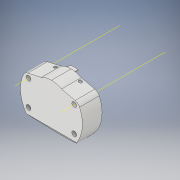
# Autodesk Inventor part: DGB_002_NewCover
Saved by Autodesk Inventor 2018 (Build 220112000, 112)
## iProperties
Created: 2020-01-12
Part Number: DGB_002_NewCover
Material: ABS Plastic
Document SubType Name: Modeling
Designer: user
Density: 1.06 g/cm^3
Appearance: Smooth - White
Mass: 38.8986 g
Surface Area: 471.13 cm^2
Volume: 36.6968 cm^3
Author: user
Autodesk Inventor part; units mm, degrees
ref_plane "YZ Plane" through (0, 0, 0) normal (1, 0, 0) x (0, 1, 0)
sketch "Sketch1" plane through (0, 0, 0) normal (0, 0, 1) x (1, 0, 0)
  line L0 (61.459706, -2.433337) -> (77.570916, 69.357275) construction
  arc A0 (77.570916, 69.357275) -> (52.904901, 108.47351) centre (45.600116, 76.532144) ccw construction
  line L1 (9.160225, 118.477636) -> (52.904901, 108.47351) construction
  arc A1 (9.160225, 118.477636) -> (-9.526433, 118.477636) centre (-0.183104, 77.6224) ccw construction
  line L2 (-9.526433, 118.477636) -> (-53.271109, 108.47351) construction
  arc A2 (-53.271109, 108.47351) -> (-77.937124, 69.357275) centre (-45.966325, 76.532144) ccw construction
  line L3 (-77.937124, 69.357275) -> (-61.825914, -2.433337) construction
  arc A3 (-61.825914, -2.433337) -> (-56.608807, -9.583273) centre (-50.983104, 0) ccw construction
  line L4 (-56.608807, -9.583273) -> (-18.828292, -31.761705) construction
  arc A4 (-18.828292, -31.761705) -> (18.462083, -31.761705) centre (-0.183104, 0) ccw construction
  line L5 (56.242599, -9.583273) -> (18.462083, -31.761705) construction
  arc A5 (56.242599, -9.583273) -> (61.459706, -2.433337) centre (50.616896, 0) ccw construction
  circle A6 centre (0, 41.9862) radius 14.2875 construction
  circle A7 centre (0, 77.6224) radius 14.2875 construction
  circle A8 centre (45.78322, 76.532144) radius 9.5631 construction
  circle A9 centre (23.8125, 0) radius 2.0193 construction
  circle A10 centre (-23.8125, 0) radius 2.0193 construction
  circle A11 centre (15.947858, 9.2075) radius 2.0193 construction
  circle A12 centre (-15.947858, 9.2075) radius 2.0193 construction
  circle A13 centre (0, -18.415) radius 2.0193 construction
  circle A14 centre (-45.78322, 51.132144) radius 2.4892 construction
  circle A15 centre (-45.78322, 101.932144) radius 2.4892 construction
  circle A16 centre (45.78322, 101.932144) radius 2.4892 construction
  circle A17 centre (45.78322, 51.132144) radius 2.4892 construction
  circle A18 centre (50.8, 0) radius 9.5758 construction
  circle A19 centre (-50.8, 0) radius 9.5758 construction
  line L6 (-3.175, 99.337246) -> (-3.175, 109.347752) construction
  arc A20 (-5.473828, 96.26646) -> (-3.175, 99.337246) centre (-6.3754, 99.337246) ccw construction
  arc A21 (-5.473828, 96.26646) -> (-18.769089, 82.650824) centre (0, 77.6224) ccw construction
  arc A22 (-21.784278, 80.279542) -> (-18.769089, 82.650824) centre (-21.860469, 83.479034) ccw construction
  line L7 (-21.784278, 80.279542) -> (-27.885438, 80.134252) construction
  arc A23 (-30.95167, 82.192597) -> (-27.885438, 80.134252) centre (-27.961629, 83.333745) ccw construction
  arc A24 (-30.95167, 82.192597) -> (-40.477461, 91.494248) centre (-45.78322, 76.532144) ccw construction
  arc A25 (-42.60822, 94.510608) -> (-40.477461, 91.494248) centre (-39.40782, 94.510608) ccw construction
  line L8 (-42.60822, 94.510608) -> (-42.60822, 95.929379) construction
  arc A26 (-41.737916, 98.123283) -> (-42.60822, 95.929379) centre (-39.40782, 95.929379) ccw construction
  arc A27 (-41.737916, 98.123283) -> (-40.233223, 102.195657) centre (-45.78322, 101.932144) ccw construction
  arc A28 (-37.749915, 105.467294) -> (-40.233223, 102.195657) centre (-37.036424, 102.34744) ccw construction
  line L9 (-7.927673, 112.287449) -> (-37.749915, 105.467294) construction
  arc A29 (-7.005934, 112.485425) -> (-7.927673, 112.287449) centre (0, 77.6224) ccw construction
  arc A30 (-3.175, 109.347752) -> (-7.005934, 112.485425) centre (-6.3754, 109.347752) ccw construction
  arc A31 (-54.866106, 101.337511) -> (-71.349124, 83.179673) centre (-45.78322, 76.532144) ccw construction
  arc A32 (-50.848233, 99.647945) -> (-54.866106, 101.337511) centre (-53.765679, 98.332246) ccw construction
  arc A33 (-50.848233, 99.647945) -> (-49.828525, 98.123283) centre (-45.78322, 101.932144) ccw construction
  arc A34 (-48.95822, 95.929379) -> (-49.828525, 98.123283) centre (-52.15862, 95.929379) ccw construction
  line L10 (-48.95822, 94.510608) -> (-48.95822, 95.929379) construction
  arc A35 (-51.088979, 91.494248) -> (-48.95822, 94.510608) centre (-52.15862, 94.510608) ccw construction
  arc A36 (-51.088979, 91.494248) -> (-60.867396, 81.480201) centre (-45.78322, 76.532144) ccw construction
  arc A37 (-63.832175, 79.278237) -> (-60.867396, 81.480201) centre (-63.908366, 82.477729) ccw construction
  line L11 (-63.832175, 79.278237) -> (-68.175525, 79.174806) construction
  arc A38 (-71.349124, 83.179673) -> (-68.175525, 79.174806) centre (-68.251716, 82.374299) ccw construction
  line L12 (-63.681003, 72.930036) -> (-68.102406, 72.824747) construction
  arc A39 (-60.614771, 70.871691) -> (-63.681003, 72.930036) centre (-63.604812, 69.730543) ccw construction
  arc A40 (-60.614771, 70.871691) -> (-51.088979, 61.57004) centre (-45.78322, 76.532144) ccw construction
  arc A41 (-48.95822, 58.55368) -> (-51.088979, 61.57004) centre (-52.15862, 58.55368) ccw construction
  line L13 (-48.95822, 57.13491) -> (-48.95822, 58.55368) construction
  arc A42 (-49.828525, 54.941005) -> (-48.95822, 57.13491) centre (-52.15862, 57.13491) ccw construction
  arc A43 (-49.828525, 54.941005) -> (-51.248421, 52.133894) centre (-45.78322, 51.132144) ccw construction
  arc A44 (-52.500008, 50.13285) -> (-51.248421, 52.133894) centre (-54.396376, 52.710901) ccw construction
  line L14 (-52.500008, 50.13285) -> (-60.545848, 44.214475) construction
  arc A45 (-62.828817, 43.615562) -> (-60.545848, 44.214475) centre (-62.442216, 46.792526) ccw construction
  arc A46 (-62.828817, 43.615562) -> (-63.126943, 43.643712) centre (-63.5, 38.1) ccw construction
  arc A47 (-66.034792, 46.136089) -> (-63.126943, 43.643712) centre (-62.912063, 46.83689) ccw construction
  line L15 (-71.148944, 68.924453) -> (-66.034792, 46.136089) construction
  arc A48 (-68.102406, 72.824747) -> (-71.148944, 68.924453) centre (-68.026215, 69.625254) ccw construction
  line L16 (-40.941493, -11.309739) -> (-15.4305, -26.285549) construction
  arc A49 (-41.887958, -6.63801) -> (-40.941493, -11.309739) centre (-39.32129, -8.549756) ccw construction
  arc A50 (-41.887958, -6.63801) -> (-40.850794, -4.949845) centre (-50.8, 0) ccw construction
  arc A51 (-37.985423, -3.175) -> (-40.850794, -4.949845) centre (-37.985423, -6.3754) ccw construction
  line L17 (-29.815266, -3.175) -> (-37.985423, -3.175) construction
  arc A52 (-27.621361, -4.045305) -> (-29.815266, -3.175) centre (-29.815266, -6.3754) ccw construction
  arc A53 (-27.621361, -4.045305) -> (-21.832221, -5.191378) centre (-23.8125, 0) ccw construction
  arc A54 (-17.715395, -7.004805) -> (-21.832221, -5.191378) centre (-20.691581, -8.181612) ccw construction
  arc A55 (-17.715395, -7.004805) -> (-7.267025, -17.609453) centre (0, 0) ccw construction
  arc A56 (-5.385714, -19.781016) -> (-7.267025, -17.609453) centre (-8.487885, -20.567842) ccw construction
  arc A57 (-5.385714, -19.781016) -> (-4.045305, -22.223861) centre (0, -18.415) ccw construction
  arc A58 (-3.175, -24.417766) -> (-4.045305, -22.223861) centre (-6.3754, -24.417766) ccw construction
  line L18 (-3.175, -26.524156) -> (-3.175, -24.417766) construction
  arc A59 (-7.123352, -29.635928) -> (-3.175, -26.524156) centre (-6.3754, -26.524156) ccw construction
  arc A60 (-15.4305, -26.285549) -> (-7.123352, -29.635928) centre (0, 0) ccw construction
  arc A61 (18.769089, 82.650824) -> (5.473828, 96.26646) centre (0, 77.6224) ccw construction
  arc A62 (3.175, 99.337246) -> (5.473828, 96.26646) centre (6.3754, 99.337246) ccw construction
  line L19 (3.175, 99.337246) -> (3.175, 109.347752) construction
  arc A63 (7.005934, 112.485425) -> (3.175, 109.347752) centre (6.3754, 109.347752) ccw construction
  arc A64 (7.927673, 112.287449) -> (7.005934, 112.485425) centre (0, 77.6224) ccw construction
  line L20 (7.927673, 112.287449) -> (37.749915, 105.467294) construction
  arc A65 (40.233223, 102.195657) -> (37.749915, 105.467294) centre (37.036424, 102.34744) ccw construction
  arc A66 (40.233223, 102.195657) -> (41.737916, 98.123283) centre (45.78322, 101.932144) ccw construction
  arc A67 (42.60822, 95.929379) -> (41.737916, 98.123283) centre (39.40782, 95.929379) ccw construction
  line L21 (42.60822, 94.510608) -> (42.60822, 95.929379) construction
  arc A68 (40.477461, 91.494248) -> (42.60822, 94.510608) centre (39.40782, 94.510608) ccw construction
  arc A69 (40.477461, 91.494248) -> (30.95167, 82.192597) centre (45.78322, 76.532144) ccw construction
  arc A70 (27.885438, 80.134252) -> (30.95167, 82.192597) centre (27.961629, 83.333745) ccw construction
  line L22 (21.784278, 80.279542) -> (27.885438, 80.134252) construction
  arc A71 (18.769089, 82.650824) -> (21.784278, 80.279542) centre (21.860469, 83.479034) ccw construction
  arc A72 (49.828525, 98.123283) -> (50.848233, 99.647945) centre (45.78322, 101.932144) ccw construction
  arc A73 (54.866106, 101.337511) -> (50.848233, 99.647945) centre (53.765679, 98.332246) ccw construction
  arc A74 (71.349124, 83.179673) -> (54.866106, 101.337511) centre (45.78322, 76.532144) ccw construction
  arc A75 (68.175525, 79.174806) -> (71.349124, 83.179673) centre (68.251716, 82.374299) ccw construction
  line L23 (63.832175, 79.278237) -> (68.175525, 79.174806) construction
  arc A76 (60.867396, 81.480201) -> (63.832175, 79.278237) centre (63.908366, 82.477729) ccw construction
  arc A77 (60.867396, 81.480201) -> (51.088979, 91.494248) centre (45.78322, 76.532144) ccw construction
  arc A78 (48.95822, 94.510608) -> (51.088979, 91.494248) centre (52.15862, 94.510608) ccw construction
  line L24 (48.95822, 94.510608) -> (48.95822, 95.929379) construction
  arc A79 (49.828525, 98.123283) -> (48.95822, 95.929379) centre (52.15862, 95.929379) ccw construction
  arc A80 (54.402179, 10.512467) -> (49.473378, 11.033029) centre (50.8, 0) ccw construction
  arc A81 (46.416616, 12.45311) -> (49.473378, 11.033029) centre (49.091311, 14.210541) ccw construction
  line L25 (46.416616, 12.45311) -> (28.364069, 39.927902) construction
  arc A82 (30.411819, 44.823724) -> (28.364069, 39.927902) centre (31.038764, 41.685333) ccw construction
  line L26 (30.411819, 44.823724) -> (40.518729, 46.842744) construction
  arc A83 (42.840615, 46.419079) -> (40.518729, 46.842744) centre (41.145674, 43.704353) ccw construction
  arc A84 (42.840615, 46.419079) -> (46.454403, 45.616582) centre (45.78322, 51.132144) ccw construction
  arc A85 (48.737373, 45.017669) -> (46.454403, 45.616582) centre (46.841005, 42.439618) ccw construction
  line L27 (48.737373, 45.017669) -> (56.783213, 39.099294) construction
  arc A86 (58.0348, 37.09825) -> (56.783213, 39.099294) centre (54.886845, 36.521243) ccw construction
  arc A87 (58.0348, 37.09825) -> (60.793794, 33.247334) centre (63.5, 38.1) ccw construction
  arc A88 (62.357749, 29.751398) -> (60.793794, 33.247334) centre (59.23502, 30.452199) ccw construction
  line L28 (62.357749, 29.751398) -> (58.562335, 12.839257) construction
  arc A89 (54.402179, 10.512467) -> (58.562335, 12.839257) centre (55.439606, 13.540058) ccw construction
  arc A90 (12.787451, 62.992128) -> (12.738922, 56.150322) centre (15.796264, 59.549712) ccw construction
  arc A91 (12.787451, 62.992128) -> (18.508462, 71.70627) centre (0, 77.6224) ccw construction
  arc A92 (21.633105, 73.931341) -> (18.508462, 71.70627) centre (21.556915, 70.731848) ccw construction
  line L29 (21.633105, 73.931341) -> (27.734266, 73.786052) construction
  arc A93 (30.699045, 71.584087) -> (27.734266, 73.786052) centre (27.658075, 70.586559) ccw construction
  arc A94 (30.699045, 71.584087) -> (40.477461, 61.57004) centre (45.78322, 76.532144) ccw construction
  arc A95 (42.60822, 58.55368) -> (40.477461, 61.57004) centre (39.40782, 58.55368) ccw construction
  line L30 (42.60822, 57.13491) -> (42.60822, 58.55368) construction
  arc A96 (41.737916, 54.941005) -> (42.60822, 57.13491) centre (39.40782, 57.13491) ccw construction
  arc A97 (41.737916, 54.941005) -> (41.255699, 54.35293) centre (45.78322, 51.132144) ccw construction
  arc A98 (39.274791, 53.069711) -> (41.255699, 54.35293) centre (38.647846, 56.208103) ccw construction
  line L31 (20.28247, 49.275686) -> (39.274791, 53.069711) construction
  arc A99 (16.828361, 50.914177) -> (20.28247, 49.275686) centre (19.655525, 52.414077) ccw construction
  arc A100 (16.828361, 50.914177) -> (12.738922, 56.150322) centre (0, 41.9862) ccw construction
  arc A101 (40.850794, -4.949845) -> (41.887958, -6.63801) centre (50.8, 0) ccw construction
  arc A102 (40.941493, -11.309739) -> (41.887958, -6.63801) centre (39.32129, -8.549756) ccw construction
  line L32 (40.941493, -11.309739) -> (15.4305, -26.285549) construction
  arc A103 (7.123352, -29.635928) -> (15.4305, -26.285549) centre (0, 0) ccw construction
  arc A104 (3.175, -26.524156) -> (7.123352, -29.635928) centre (6.3754, -26.524156) ccw construction
  line L33 (3.175, -26.524156) -> (3.175, -24.417766) construction
  arc A105 (4.045305, -22.223861) -> (3.175, -24.417766) centre (6.3754, -24.417766) ccw construction
  arc A106 (4.045305, -22.223861) -> (5.385714, -19.781016) centre (0, -18.415) ccw construction
  arc A107 (7.267025, -17.609453) -> (5.385714, -19.781016) centre (8.487885, -20.567842) ccw construction
  arc A108 (7.267025, -17.609453) -> (17.715395, -7.004805) centre (0, 0) ccw construction
  arc A109 (21.832221, -5.191378) -> (17.715395, -7.004805) centre (20.691581, -8.181612) ccw construction
  arc A110 (21.832221, -5.191378) -> (27.621361, -4.045305) centre (23.8125, 0) ccw construction
  arc A111 (29.815266, -3.175) -> (27.621361, -4.045305) centre (29.815266, -6.3754) ccw construction
  line L34 (29.815266, -3.175) -> (37.985423, -3.175) construction
  arc A112 (40.850794, -4.949845) -> (37.985423, -3.175) centre (37.985423, -6.3754) ccw construction
  arc A113 (51.088979, 61.57004) -> (60.614771, 70.871691) centre (45.78322, 76.532144) ccw construction
  arc A114 (63.681003, 72.930036) -> (60.614771, 70.871691) centre (63.604812, 69.730543) ccw construction
  line L35 (63.681003, 72.930036) -> (68.102406, 72.824747) construction
  arc A115 (71.148944, 68.924453) -> (68.102406, 72.824747) centre (68.026215, 69.625254) ccw construction
  line L36 (71.148944, 68.924453) -> (66.034792, 46.136089) construction
  arc A116 (63.126943, 43.643712) -> (66.034792, 46.136089) centre (62.912063, 46.83689) ccw construction
  arc A117 (63.126943, 43.643712) -> (62.828817, 43.615562) centre (63.5, 38.1) ccw construction
  arc A118 (60.545848, 44.214475) -> (62.828817, 43.615562) centre (62.442216, 46.792526) ccw construction
  line L37 (52.500008, 50.13285) -> (60.545848, 44.214475) construction
  arc A119 (51.248421, 52.133894) -> (52.500008, 50.13285) centre (54.396376, 52.710901) ccw construction
  arc A120 (51.248421, 52.133894) -> (49.828525, 54.941005) centre (45.78322, 51.132144) ccw construction
  arc A121 (48.95822, 57.13491) -> (49.828525, 54.941005) centre (52.15862, 57.13491) ccw construction
  line L38 (48.95822, 57.13491) -> (48.95822, 58.55368) construction
  arc A122 (51.088979, 61.57004) -> (48.95822, 58.55368) centre (52.15862, 58.55368) ccw construction
  arc A123 (11.616722, 15.098155) -> (8.733861, 16.929919) centre (0, 0) ccw construction
  arc A124 (8.733861, 25.056281) -> (8.733861, 16.929919) centre (10.829988, 20.9931) ccw construction
  arc A125 (8.733861, 25.056281) -> (17.800734, 35.201189) centre (0, 41.9862) ccw construction
  arc A126 (23.465953, 35.818739) -> (17.800734, 35.201189) centre (20.791257, 34.061308) ccw construction
  line L39 (41.109681, 8.966143) -> (23.465953, 35.818739) construction
  arc A127 (41.199833, 5.596826) -> (41.109681, 8.966143) centre (38.434985, 7.208711) ccw construction
  arc A128 (41.199833, 5.596826) -> (40.850794, 4.949845) centre (50.8, 0) ccw construction
  arc A129 (37.985423, 3.175) -> (40.850794, 4.949845) centre (37.985423, 6.3754) ccw construction
  line L40 (29.815266, 3.175) -> (37.985423, 3.175) construction
  arc A130 (27.621361, 4.045305) -> (29.815266, 3.175) centre (29.815266, 6.3754) ccw construction
  arc A131 (27.621361, 4.045305) -> (24.369611, 5.528249) centre (23.8125, 0) ccw construction
  arc A132 (21.495224, 8.893427) -> (24.369611, 5.528249) centre (24.690507, 8.712521) ccw construction
  arc A133 (21.495224, 8.893427) -> (14.438006, 14.554673) centre (15.947858, 9.2075) ccw construction
  arc A134 (11.616722, 15.098155) -> (14.438006, 14.554673) centre (13.568331, 17.634645) ccw construction
  line L41 (-21.633105, 73.931341) -> (-27.734266, 73.786052) construction
  arc A135 (-18.508462, 71.70627) -> (-21.633105, 73.931341) centre (-21.556915, 70.731848) ccw construction
  arc A136 (-18.508462, 71.70627) -> (-12.787451, 62.992128) centre (0, 77.6224) ccw construction
  arc A137 (-12.738922, 56.150322) -> (-12.787451, 62.992128) centre (-15.796264, 59.549712) ccw construction
  arc A138 (-12.738922, 56.150322) -> (-16.828361, 50.914177) centre (0, 41.9862) ccw construction
  arc A139 (-20.28247, 49.275686) -> (-16.828361, 50.914177) centre (-19.655525, 52.414077) ccw construction
  line L42 (-20.28247, 49.275686) -> (-39.274791, 53.069711) construction
  arc A140 (-41.255699, 54.35293) -> (-39.274791, 53.069711) centre (-38.647846, 56.208103) ccw construction
  arc A141 (-41.255699, 54.35293) -> (-41.737916, 54.941005) centre (-45.78322, 51.132144) ccw construction
  arc A142 (-42.60822, 57.13491) -> (-41.737916, 54.941005) centre (-39.40782, 57.13491) ccw construction
  line L43 (-42.60822, 57.13491) -> (-42.60822, 58.55368) construction
  arc A143 (-40.477461, 61.57004) -> (-42.60822, 58.55368) centre (-39.40782, 58.55368) ccw construction
  arc A144 (-40.477461, 61.57004) -> (-30.699045, 71.584087) centre (-45.78322, 76.532144) ccw construction
  arc A145 (-27.734266, 73.786052) -> (-30.699045, 71.584087) centre (-27.658075, 70.586559) ccw construction
  arc A146 (-8.733861, 16.929919) -> (-8.733861, 25.056281) centre (-10.829988, 20.9931) ccw construction
  arc A147 (-8.733861, 16.929919) -> (-11.616722, 15.098155) centre (0, 0) ccw construction
  arc A148 (-14.438006, 14.554673) -> (-11.616722, 15.098155) centre (-13.568331, 17.634645) ccw construction
  arc A149 (-14.438006, 14.554673) -> (-21.495224, 8.893427) centre (-15.947858, 9.2075) ccw construction
  arc A150 (-24.369611, 5.528249) -> (-21.495224, 8.893427) centre (-24.690507, 8.712521) ccw construction
  arc A151 (-24.369611, 5.528249) -> (-27.621361, 4.045305) centre (-23.8125, 0) ccw construction
  arc A152 (-29.815266, 3.175) -> (-27.621361, 4.045305) centre (-29.815266, 6.3754) ccw construction
  line L44 (-29.815266, 3.175) -> (-37.985423, 3.175) construction
  arc A153 (-40.850794, 4.949845) -> (-37.985423, 3.175) centre (-37.985423, 6.3754) ccw construction
  arc A154 (-40.850794, 4.949845) -> (-41.199833, 5.596826) centre (-50.8, 0) ccw construction
  arc A155 (-41.109681, 8.966143) -> (-41.199833, 5.596826) centre (-38.434985, 7.208711) ccw construction
  line L45 (-41.109681, 8.966143) -> (-23.465953, 35.818739) construction
  arc A156 (-17.800734, 35.201189) -> (-23.465953, 35.818739) centre (-20.791257, 34.061308) ccw construction
  arc A157 (-17.800734, 35.201189) -> (-8.733861, 25.056281) centre (0, 41.9862) ccw construction
  line L46 (-46.416616, 12.45311) -> (-28.364069, 39.927902) construction
  arc A158 (-49.473378, 11.033029) -> (-46.416616, 12.45311) centre (-49.091311, 14.210541) ccw construction
  arc A159 (-49.473378, 11.033029) -> (-54.402179, 10.512467) centre (-50.8, 0) ccw construction
  arc A160 (-58.562335, 12.839257) -> (-54.402179, 10.512467) centre (-55.439606, 13.540058) ccw construction
  line L47 (-62.357749, 29.751398) -> (-58.562335, 12.839257) construction
  arc A161 (-60.793794, 33.247334) -> (-62.357749, 29.751398) centre (-59.23502, 30.452199) ccw construction
  arc A162 (-60.793794, 33.247334) -> (-58.0348, 37.09825) centre (-63.5, 38.1) ccw construction
  arc A163 (-56.783213, 39.099294) -> (-58.0348, 37.09825) centre (-54.886845, 36.521243) ccw construction
  line L48 (-48.737373, 45.017669) -> (-56.783213, 39.099294) construction
  arc A164 (-46.454403, 45.616582) -> (-48.737373, 45.017669) centre (-46.841005, 42.439618) ccw construction
  arc A165 (-46.454403, 45.616582) -> (-42.840615, 46.419079) centre (-45.78322, 51.132144) ccw construction
  arc A166 (-40.518729, 46.842744) -> (-42.840615, 46.419079) centre (-41.145674, 43.704353) ccw construction
  line L49 (-30.411819, 44.823724) -> (-40.518729, 46.842744) construction
  arc A167 (-28.364069, 39.927902) -> (-30.411819, 44.823724) centre (-31.038764, 41.685333) ccw construction
  circle A168 centre (63.5, 38.1) radius 2.4892 construction
  circle A169 centre (0, 0) radius 14.2875 construction
  circle A170 centre (-63.5, 38.1) radius 2.4892 construction
  circle A171 centre (-45.78322, 76.532144) radius 9.5631 construction
  circle A172 centre (0, 77.6224) radius 39.37 construction
  circle A173 centre (0, 41.9862) radius 26.67 construction
  arc A174 (-53.271109, 108.47351) -> (-77.937124, 69.357275) centre (-45.966325, 76.532144) ccw construction
  line L50 (0, 157.262223) -> (0, -96.319817) construction
  circle A175 centre (-45.78322, 76.532144) radius 8.89 construction
  arc A176 (-56.25745, 102.583954) -> (0, 10.061701) centre (3.886504, 75.789444) ccw
  arc A177 (-47.487931, 109.796086) -> (-56.25745, 102.583954) centre (-44.656619, 97.415711) ccw
  line L51 (-47.487931, 109.796086) -> (-20.215243, 116.033174)
  arc A178 (0, 121.113165) -> (-20.215243, 116.033174) centre (0.183104, 77.6224) ccw
  arc A179 (0, 10.061701) -> (56.25745, 102.583954) centre (-3.886504, 75.789444) ccw
  arc A180 (56.25745, 102.583954) -> (47.487931, 109.796086) centre (44.656619, 97.415711) ccw
  line L52 (47.487931, 109.796086) -> (20.215243, 116.033174)
  arc A181 (20.215243, 116.033174) -> (0, 121.113165) centre (-0.183104, 77.6224) ccw
  line L53 (-19.654425, 114.532945) -> (-47.134017, 108.248539)
  arc A182 (-47.134017, 108.248539) -> (-54.807346, 101.937924) centre (-44.656619, 97.415711) ccw
  arc A183 (-54.807346, 101.937924) -> (0, 11.652043) centre (3.886504, 75.789444) ccw
  arc A184 (0, 11.652043) -> (54.807346, 101.937924) centre (-3.886504, 75.789444) ccw
  arc A185 (54.807346, 101.937924) -> (47.134017, 108.248539) centre (44.656619, 97.415711) ccw
  line L54 (47.134017, 108.248539) -> (19.654425, 114.532945)
  arc A186 (19.654425, 114.532945) -> (0, 119.52565) centre (-0.183104, 77.6224) ccw
  arc A187 (0, 119.52565) -> (-19.654425, 114.532945) centre (0.183104, 77.6224) ccw
  point P0 (0, 0)
  dimension "d0" = 78.74
  dimension "d1" = 53.34
  dimension "d9" = 17.78
  dimension "d10" = 12.7
  dimension "d11" = 0
  dimension "d12" = 0
  dimension "d13" = 1.5875
  dimension "d16" = 43.49115
  constraints: 334 point on circle, 188 centre point, 110 end point, 6 symmetric about line, 3 point on line, 2 coincident, 1 concentric, 1 tangent, 1 vertical, 12 other
  measures "d0" diameter of A172
  measures "d1" diameter of A173
  measures "d9" diameter of A175
  measures "d10" radius of A177
  measures "d11" distance from line of L50 A169.centre
  measures "d12" distance from line of point (0, 0) L50
  measures "d13" distance between parallel lines of L51 L53
  measures "d16" radius of A181
sketch "Sketch1 outline for Extrusion1" plane through (0, 0, 0) normal (0, 0, 1) x (1, 0, 0)
  arc A0 (0, 10.061701) -> (-56.25745, 102.583954) centre (3.886504, 75.789444) cw
  arc A1 (56.25745, 102.583954) -> (0, 10.061701) centre (-3.886504, 75.789444) cw
  arc A2 (-56.25745, 102.583954) -> (-47.487931, 109.796086) centre (-44.656619, 97.415711) cw
  arc A3 (47.487931, 109.796086) -> (56.25745, 102.583954) centre (44.656619, 97.415711) cw
  line L0 (-47.487931, 109.796086) -> (-20.215243, 116.033174)
  line L1 (20.215243, 116.033174) -> (47.487931, 109.796086)
  arc A4 (-20.215243, 116.033174) -> (0, 121.113165) centre (0.183104, 77.6224) cw
  arc A5 (0, 121.113165) -> (20.215243, 116.033174) centre (-0.183104, 77.6224) cw
  arc A6 (0, 119.52565) -> (-19.654425, 114.532945) centre (0.183104, 77.6224) ccw
  line L2 (-19.654425, 114.532945) -> (-47.134017, 108.248539)
  arc A7 (-47.134017, 108.248539) -> (-54.807346, 101.937924) centre (-44.656619, 97.415711) ccw
  arc A8 (-54.807346, 101.937924) -> (0, 11.652043) centre (3.886504, 75.789444) ccw
  arc A9 (0, 11.652043) -> (54.807346, 101.937924) centre (-3.886504, 75.789444) ccw
  arc A10 (54.807346, 101.937924) -> (47.134017, 108.248539) centre (44.656619, 97.415711) ccw
  line L3 (47.134017, 108.248539) -> (19.654425, 114.532945)
  arc A11 (19.654425, 114.532945) -> (0, 119.52565) centre (-0.183104, 77.6224) ccw
extrude "Extrusion1" add sketch "Sketch1 outline for Extrusion1" along normal blind 37.7952
sketch "Sketch3" plane through (0, 0, 37.7952) normal (0, 0, 1) x (1, 0, 0)
  arc A0 (0, 119.52565) -> (-19.654425, 114.532945) centre (0.183104, 77.6224) ccw
  arc A1 (19.654425, 114.532945) -> (0, 119.52565) centre (-0.183104, 77.6224) ccw
  line L0 (19.654425, 114.532945) -> (47.134017, 108.248539)
  arc A2 (54.807346, 101.937924) -> (47.134017, 108.248539) centre (44.656619, 97.415711) ccw
  arc A3 (0, 11.652043) -> (54.807346, 101.937924) centre (-3.886504, 75.789444) ccw
  arc A4 (-54.807346, 101.937924) -> (0, 11.652043) centre (3.886504, 75.789444) ccw
  arc A5 (-47.134017, 108.248539) -> (-54.807346, 101.937924) centre (-44.656619, 97.415711) ccw
  line L1 (-47.134017, 108.248539) -> (-19.654425, 114.532945)
  arc A6 (-56.25745, 102.583954) -> (0, 10.061701) centre (3.886504, 75.789444) ccw
  arc A7 (0, 10.061701) -> (56.25745, 102.583954) centre (-3.886504, 75.789444) ccw
  arc A8 (56.25745, 102.583954) -> (47.487931, 109.796086) centre (44.656619, 97.415711) ccw
  line L2 (47.487931, 109.796086) -> (20.215243, 116.033174)
  arc A9 (20.215243, 116.033174) -> (0, 121.113165) centre (-0.183104, 77.6224) ccw
  arc A10 (0, 121.113165) -> (-20.215243, 116.033174) centre (0.183104, 77.6224) ccw
  line L3 (-20.215243, 116.033174) -> (-47.487931, 109.796086)
  arc A11 (-47.487931, 109.796086) -> (-56.25745, 102.583954) centre (-44.656619, 97.415711) ccw
  point P0 (0, 0)
sketch "Sketch3 outline for Extrusion3" plane through (0, 0, 37.7952) normal (0, 0, 1) x (1, 0, 0)
  arc A0 (-47.487931, 109.796086) -> (-56.25745, 102.583954) centre (-44.656619, 97.415711) ccw
  line L0 (-20.215243, 116.033174) -> (-47.487931, 109.796086)
  arc A1 (0, 121.113165) -> (-20.215243, 116.033174) centre (0.183104, 77.6224) ccw
  arc A2 (20.215243, 116.033174) -> (0, 121.113165) centre (-0.183104, 77.6224) ccw
  line L1 (47.487931, 109.796086) -> (20.215243, 116.033174)
  arc A3 (56.25745, 102.583954) -> (47.487931, 109.796086) centre (44.656619, 97.415711) ccw
  arc A4 (0, 10.061701) -> (56.25745, 102.583954) centre (-3.886504, 75.789444) ccw
  arc A5 (-56.25745, 102.583954) -> (0, 10.061701) centre (3.886504, 75.789444) ccw
extrude "Extrusion3" add sketch "Sketch3 outline for Extrusion3" along normal blind 1.5875
sketch "Sketch4" plane through (0, 0, 0) normal (0, 0, -1) x (-1, 0, 0)
  arc A0 (19.654425, 114.532945) -> (0, 119.52565) centre (-0.183104, 77.6224) ccw
  line L0 (19.654425, 114.532945) -> (47.134017, 108.248539)
  arc A1 (54.807346, 101.937924) -> (47.134017, 108.248539) centre (44.656619, 97.415711) ccw
  arc A2 (0, 11.652043) -> (54.807346, 101.937924) centre (-3.886504, 75.789444) ccw
  arc A3 (-54.807346, 101.937924) -> (0, 11.652043) centre (3.886504, 75.789444) ccw
  arc A4 (-47.134017, 108.248539) -> (-54.807346, 101.937924) centre (-44.656619, 97.415711) ccw
  line L1 (-47.134017, 108.248539) -> (-19.654425, 114.532945)
  arc A5 (0, 119.52565) -> (-19.654425, 114.532945) centre (0.183104, 77.6224) ccw
  arc A6 (0, 10.061701) -> (56.25745, 102.583954) centre (-3.886504, 75.789444) ccw
  arc A7 (56.25745, 102.583954) -> (47.487931, 109.796086) centre (44.656619, 97.415711) ccw
  line L2 (47.487931, 109.796086) -> (20.215243, 116.033174)
  arc A8 (20.215243, 116.033174) -> (0, 121.113165) centre (-0.183104, 77.6224) ccw
  arc A9 (0, 121.113165) -> (-20.215243, 116.033174) centre (0.183104, 77.6224) ccw
  line L3 (-20.215243, 116.033174) -> (-47.487931, 109.796086)
  arc A10 (-47.487931, 109.796086) -> (-56.25745, 102.583954) centre (-44.656619, 97.415711) ccw
  arc A11 (-56.25745, 102.583954) -> (0, 10.061701) centre (3.886504, 75.789444) ccw
  line L4 (-7.368181, 118.840041) -> (-7.722095, 120.387588)
  line L5 (0, 128.491917) -> (0, 111.62122) construction
  line L6 (7.368181, 118.840041) -> (7.722095, 120.387588)
  arc A12 (7.722095, 120.387588) -> (-7.722095, 120.387588) centre (0, 79.658377) ccw
  arc A13 (7.368181, 118.840041) -> (-7.368181, 118.840041) centre (0, 79.590206) ccw
  point P0 (0, 0)
  dimension "d17" = 1.5875
  constraints: 7 point on circle, 6 end point, 2 centre point, 2 symmetric about line, 1 vertical
  measures "d17" distance of L4.start L4.end
sketch "Sketch4 outline for Extrusion4" plane through (0, 0, 0) normal (0, 0, -1) x (-1, 0, 0)
  arc A0 (-7.368181, 118.840041) -> (0, 119.52565) centre (0, 79.590206) cw
  line L0 (-7.722095, 120.387588) -> (-7.368181, 118.840041)
  arc A1 (0, 121.113165) -> (-7.722095, 120.387588) centre (0, 79.658377) ccw
  arc A2 (7.722095, 120.387588) -> (0, 121.113165) centre (0, 79.658377) ccw
  line L1 (7.368181, 118.840041) -> (7.722095, 120.387588)
  arc A3 (0, 119.52565) -> (7.368181, 118.840041) centre (0, 79.590206) cw
extrude "Extrusion4" add sketch "Sketch4 outline for Extrusion4" along normal blind 6.35
sketch "Sketch5" plane through (0, 0, 0) normal (1, 0, 0) x (0, 1, 0)
  line L0 (102.583954, 0) -> (10.061701, 0)
  line L1 (102.583954, 0) -> (102.583954, 39.3827)
  line L2 (10.061701, 39.3827) -> (102.583954, 39.3827)
  line L3 (10.061701, 0) -> (10.061701, 39.3827)
  line L4 (10.061701, 11.43) -> (40.541701, 39.3827)
  line L5 (40.541701, 39.3827) -> (20.303879, 61.450294)
  line L6 (20.303879, 61.450294) -> (-10.176121, 33.497594)
  line L7 (-10.176121, 33.497594) -> (10.061701, 11.43)
  line L8 (10.061701, 39.3827) -> (74.252437, 39.3827)
  line L9 (74.252437, 39.3827) -> (74.252437, 49.214777)
  line L10 (74.252437, 49.214777) -> (10.061701, 49.214777)
  line L11 (10.061701, 49.214777) -> (10.061701, 39.3827)
  line L12 (10.061701, 0) -> (10.061701, 39.3827)
  line L13 (10.061701, 39.3827) -> (-1.205243, 39.3827)
  line L14 (-1.205243, 39.3827) -> (-1.205243, -1.693974)
  line L15 (-1.205243, -1.693974) -> (10.061701, -1.693974)
  line L16 (10.061701, -1.693974) -> (10.061701, 39.3827)
  point P0 (0, 0)
  dimension "d20" = 11.43
  dimension "d21" = 30.48
  constraints: 24 end point, 6 parallel, 3 perpendicular, 2 horizontal, 2 point on line
  measures "d20" distance from line of L0 L4.start
  measures "d21" distance from line of L3 L4.end
sketch "Sketch5 outline for Extrusion5" plane through (0, 0, 0) normal (1, 0, 0) x (0, 1, 0)
  line L0 (10.061701, 11.43) -> (40.541701, 39.3827)
  line L1 (40.541701, 39.3827) -> (74.252437, 39.3827)
  line L2 (74.252437, 39.3827) -> (74.252437, 49.214777)
  line L3 (74.252437, 49.214777) -> (31.524867, 49.214777)
  line L4 (31.524867, 49.214777) -> (20.303879, 61.450294)
  line L5 (20.303879, 61.450294) -> (-10.176121, 33.497594)
  line L6 (-10.176121, 33.497594) -> (-1.205243, 23.715628)
  line L7 (-1.205243, 23.715628) -> (-1.205243, -1.693974)
  line L8 (-1.205243, -1.693974) -> (10.061701, -1.693974)
  line L9 (10.061701, -1.693974) -> (10.061701, 11.43)
extrude "Extrusion5" cut sketch "Sketch5 outline for Extrusion5" along normal mid plane 254
ref_plane "Work Plane1" through (0, 40.541701, 39.3827) normal (0, -0.7370012, -0.6758915) x (1, 0, 0)
sketch "Sketch6" plane through (0, 40.541701, 39.3827) normal (0, -0.7370012, -0.6758915) x (1, 0, 0)
  line L0 (-51.726782, 0) -> (51.726782, 0)
  line L1 (-51.726782, 0) -> (51.726782, 0)
  line L2 (51.726782, 0) -> (51.726782, 1.5875)
  line L3 (51.726782, 1.5875) -> (-51.726782, 1.5875)
  line L4 (-51.726782, 1.5875) -> (-51.726782, 0)
  point P0 (0, -1.623305)
  dimension "d25" = 1.5875
  constraints: 8 end point, 2 parallel, 1 horizontal, 1 perpendicular
  measures "d25" distance of L1.end L2.end
sketch "Sketch6 outline for Extrusion6" plane through (0, 40.541701, 39.3827) normal (0, -0.7370012, -0.6758915) x (1, 0, 0)
  line L0 (-51.726782, 1.5875) -> (-51.726782, 0)
  line L1 (51.726782, 1.5875) -> (-51.726782, 1.5875)
  line L2 (51.726782, 0) -> (51.726782, 1.5875)
  line L3 (-51.726782, 0) -> (51.726782, 0)
extrude "Extrusion6" add sketch "Sketch6 outline for Extrusion6" along normal blind 43.18
sketch "Sketch7" plane through (-51.726782, 40.541701, 39.3827) normal (-1, 0, 0) x (0, -0.6758915, 0.7370012)
  line L0 (-2.844297, -43.965245) -> (3.166329, -38.452999)
  line L1 (3.166329, -38.452999) -> (6.493214, -42.080679)
  line L2 (6.493214, -42.080679) -> (0.482587, -47.592924)
  line L3 (0.482587, -47.592924) -> (-2.844297, -43.965245)
  line L4 (0, -41.356787) -> (0, 0)
  line L5 (-41.93383, 45.725212) -> (0, 0)
  line L6 (-70.958926, 19.106781) -> (-41.93383, 45.725212)
  line L7 (-8.423923, -49.082227) -> (-70.958926, 19.106781)
  line L8 (-8.423923, -49.082227) -> (0, -41.356787)
  line L9 (-8.423923, -49.082227) -> (0, -41.356787)
  line L10 (-3.768096, 4.108782) -> (8.587457, -9.363879)
  line L11 (8.587457, -9.363879) -> (19.596125, 0.731987)
  line L12 (19.596125, 0.731987) -> (7.240573, 14.204648)
  line L13 (7.240573, 14.204648) -> (-3.768096, 4.108782)
  point P0 (-1.623305, -56.497712)
  constraints: 16 end point, 4 parallel, 2 collinear, 2 perpendicular, 1 point on line
sketch "Sketch7 outline for Extrusion7" plane through (-51.726782, 40.541701, 39.3827) normal (-1, 0, 0) x (0, -0.6758915, 0.7370012)
  line L0 (-2.844297, -43.965245) -> (3.166329, -38.452999)
  line L1 (3.166329, -38.452999) -> (6.493214, -42.080679)
  line L2 (6.493214, -42.080679) -> (0.482587, -47.592924)
  line L3 (0.482587, -47.592924) -> (-2.844297, -43.965245)
  line L4 (7.240573, 14.204648) -> (-3.768096, 4.108782)
  line L5 (19.596125, 0.731987) -> (7.240573, 14.204648)
  line L6 (8.587457, -9.363879) -> (19.596125, 0.731987)
  line L7 (-3.768096, 4.108782) -> (8.587457, -9.363879)
extrude "Extrusion7" cut sketch "Sketch7 outline for Extrusion7" along normal mid plane 254
sketch "Sketch8" plane through (0, 0, 0) normal (0, 0, -1) x (-1, 0, 0)
  line L0 (0, 10.061701) -> (51.726782, 10.061701)
  line L1 (51.726782, 40.541701) -> (51.726782, 10.061701)
  arc A0 (0, 10.061701) -> (51.726782, 40.541701) centre (-3.886504, 75.789444) ccw
  line L2 (-51.726782, 10.061701) -> (0, 10.061701)
  arc A1 (-51.726782, 40.541701) -> (0, 10.061701) centre (3.886504, 75.789444) ccw
  line L3 (-51.726782, 40.541701) -> (-51.726782, 10.061701)
  point P0 (0, 0)
sketch "Sketch8 outline for Extrusion8" plane through (0, 0, 0) normal (0, 0, -1) x (-1, 0, 0)
  line L0 (-51.726782, 40.541701) -> (-51.726782, 10.061701)
  arc A0 (0, 10.061701) -> (-51.726782, 40.541701) centre (3.886504, 75.789444) cw
  line L1 (-51.726782, 10.061701) -> (0, 10.061701)
  arc A1 (51.726782, 40.541701) -> (0, 10.061701) centre (-3.886504, 75.789444) cw
  line L2 (51.726782, 10.061701) -> (51.726782, 40.541701)
  line L3 (0, 10.061701) -> (51.726782, 10.061701)
extrude "Extrusion8" cut sketch "Sketch8 outline for Extrusion8" against normal blind 254
sketch "Sketch9" plane through (0, 0, 39.3827) normal (0, 0, 1) x (1, 0, 0)
  line L0 (0, 145.335797) -> (0, -24.222633)
  line L1 (-86.73846, 0) -> (86.73846, 0)
  point P0 (0, 0)
  point P1 (-45.7708, 51.1302)
  point P2 (-45.7708, 101.9302)
  point P3 (45.7708, 51.1302)
  point P4 (45.7708, 101.9302)
  dimension "d32" = 45.7708
  dimension "d33" = 45.7708
  dimension "d34" = 51.1302
  dimension "d35" = 101.9302
  constraints: 2 symmetric about line
  measures "d32" distance from line of L0 point (-45.771, 51.13)
  measures "d33" distance from line of L0 point (-45.771, 101.93)
  measures "d34" distance from line of point (-45.771, 51.13) L1
  measures "d35" distance from line of point (-45.771, 101.93) L1
hole "Hole1" at (-45.7708, 51.1302, 39.3827) at (-45.7708, 101.9302, 39.3827) at (45.7708, 51.1302, 39.3827) at (45.7708, 101.9302, 39.3827) direction (0, 0, -1) diameter 9.5504 end through all
sketch "Sketch10" plane through (0, 0, 37.7952) normal (0, 0, -1) x (-1, 0, 0)
  circle A0 centre (-45.7708, 51.1302) radius 4.7752
  circle A1 centre (45.7708, 51.1302) radius 4.7752
  circle A2 centre (45.7708, 101.9302) radius 4.7752
  circle A3 centre (-45.7708, 101.9302) radius 4.7752
  line L0 (-48.661392, 38.81067) -> (48.661392, 38.81067)
  arc A4 (48.661392, 38.81067) -> (54.807346, 101.937924) centre (-3.886504, 75.789444) ccw
  arc A5 (54.807346, 101.937924) -> (47.134017, 108.248539) centre (44.656619, 97.415711) ccw
  line L1 (47.134017, 108.248539) -> (19.654425, 114.532945)
  arc A6 (19.654425, 114.532945) -> (0, 119.52565) centre (-0.183104, 77.6224) ccw
  arc A7 (0, 119.52565) -> (-19.654425, 114.532945) centre (0.183104, 77.6224) ccw
  line L2 (-19.654425, 114.532945) -> (-47.134017, 108.248539)
  arc A8 (-47.134017, 108.248539) -> (-54.807346, 101.937924) centre (-44.656619, 97.415711) ccw
  arc A9 (-54.807346, 101.937924) -> (-48.661392, 38.81067) centre (3.886504, 75.789444) ccw
  circle A10 centre (-45.7708, 51.1302) radius 6.3627
  circle A11 centre (-45.7708, 101.9302) radius 6.3627
  circle A12 centre (45.7708, 101.9302) radius 6.3627
  circle A13 centre (45.7708, 51.1302) radius 6.3627
  point P0 (0, 0)
  dimension "d43" = 1.5875
  dimension "d44" = 1.5875
  dimension "d45" = 1.5875
  dimension "d46" = 1.5875
  constraints: 4 centre point
  measures "d43" radial gap between concentric circles of A0 A10
  measures "d44" radial gap between concentric circles of A3 A11
  measures "d45" radial gap between concentric circles of A2 A12
  measures "d46" radial gap between concentric circles of A1 A13
sketch "Sketch10 outline for Extrusion9" plane through (0, 0, 37.7952) normal (0, 0, -1) x (-1, 0, 0)
  circle A0 centre (-45.7708, 51.1302) radius 6.3627
  circle A1 centre (-45.7708, 51.1302) radius 4.7752
  circle A2 centre (-45.7708, 101.9302) radius 6.3627
  circle A3 centre (-45.7708, 101.9302) radius 4.7752
  circle A4 centre (45.7708, 101.9302) radius 6.3627
  circle A5 centre (45.7708, 101.9302) radius 4.7752
  circle A6 centre (45.7708, 51.1302) radius 6.3627
  circle A7 centre (45.7708, 51.1302) radius 4.7752
extrude "Extrusion9" add sketch "Sketch10 outline for Extrusion9" along normal blind 6.35
sketch "Sketch11" plane through (-47.487931, 109.796086, 39.3827) normal (-0.2229379, 0.9748326, 0) x (0.9748326, 0.2229379, 0)
  line L0 (48.461874, 39.3827) -> (48.461874, 1.5875)
  line L1 (0, 39.3827) -> (27.97679, 39.3827)
  point P0 (21.815072, 39.3827)
  point P1 (23.061874, 33.0327)
  dimension "d49" = 25.4
  dimension "d57" = 6.35
  measures "d49" distance from line of L0 point (23.062, 33.033)
  measures "d57" distance from line of L1 point (23.062, 33.033)
hole "Hole2" at (-25.006463, 114.937453, 6.35) direction (0.2229379, -0.9748326, 0) diameter 6.35 depth 25.4 tip angle 118
mirror "Mirror1" about plane through (0, 0, 0) normal (1, 0, 0) of "Hole2"
sketch "Sketch12" plane through (0, 0, 0) normal (0, 0, -1) x (-1, 0, 0)
  line L0 (22.86, 7.033928) -> (-22.86, 7.033928)
  line L1 (-22.86, 7.033928) -> (-22.86, 32.433928)
  line L2 (-22.86, 32.433928) -> (22.86, 32.433928)
  line L3 (22.86, 32.433928) -> (22.86, 7.033928)
  line L4 (0, -24.222633) -> (0, 145.335797)
  point P0 (0, 0)
  dimension "d58" = 22.86
  dimension "d59" = 22.86
  dimension "d62" = 25.4
  constraints: 8 end point, 2 parallel, 1 horizontal, 1 perpendicular
  measures "d58" distance between parallel lines of L4 L1
  measures "d59" distance between parallel lines of L4 L3
  measures "d62" distance of L2.end L0.start
sketch "Sketch12 outline for Extrusion10" plane through (0, 0, 0) normal (0, 0, -1) x (-1, 0, 0)
  line L0 (22.86, 7.033928) -> (-22.86, 7.033928)
  line L1 (-22.86, 7.033928) -> (-22.86, 32.433928)
  line L2 (-22.86, 32.433928) -> (22.86, 32.433928)
  line L3 (22.86, 32.433928) -> (22.86, 7.033928)
extrude "Extrusion10" cut sketch "Sketch12 outline for Extrusion10" against normal blind 5.08
ref_plane "Work Plane2" through (-45.7708, 101.9302, -133.180657) normal (0, 1, 0) x (0, 0, 1)
sketch "Sketch13" plane through (0, 0, 0) normal (0, 1, 0) x (-1, 0, 0)
  line L0 (22.86, 0) -> (61.956043, 0)
  line L1 (-61.956043, 0) -> (-22.86, 0)
  point P0 (0, 0)
  point P1 (-41.275, 6.35)
  point P2 (41.275, 6.35)
  point P3 (56.25745, 0)
  point P4 (-56.25745, 0)
  dimension "d63" = 6.35
  dimension "d64" = 6.35
  dimension "d65" = 41.275
  dimension "d66" = 41.275
  measures "d63" distance from line of L0 point (41.275, 6.35)
  measures "d64" distance from line of L1 point (-41.275, 6.35)
  measures "d65" horizontal distance of point (41.275, 6.35) point (0, 0)
  measures "d66" horizontal distance of point (-41.275, 6.35) point (0, 0)
hole "Hole3" at (41.275, 0, 6.35) at (-41.275, 0, 6.35) direction (0, 1, 0) diameter 6.35 depth 76.2 tip angle 118
equation "\"d33\" = d32"
equation "\"d59\" = d58"
equation "\"d64\" = d63"
equation "\"d66\" = d65"
body "Solid1"
